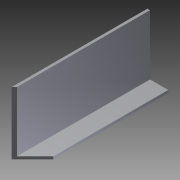
# Autodesk Inventor part: frame corner L 1 by 3
Saved by Autodesk Inventor 2012 (Build 160160000, 160)
## iProperties
Created: 2013-08-08
Part Number: frame corner L 1 by 3
Material: Default
Document SubType Name: Modeling
Designer: Bryce
Density: 1 g/cm^3
Author: Bryce
Autodesk Inventor part; units mm, degrees
ref_plane "YZ Plane" through (0, 0, 0) normal (1, 0, 0) x (0, 1, 0)
ref_plane "XZ Plane" through (0, 0, 0) normal (0, 1, 0) x (-1, 0, 0)
ref_plane "XY Plane" through (0, 0, 0) normal (0, 0, 1) x (1, 0, 0)
sketch "Sketch1" plane through (0, 0, 0) normal (0, 0, 1) x (1, 0, 0)
  line L0 (0, 0) -> (25.4, 0)
  line L1 (25.4, 0) -> (25.4, 3.175)
  line L2 (3.175, 76.2) -> (0, 76.2)
  line L3 (0, 76.2) -> (0, 0)
  line L4 (3.175, 3.175) -> (25.4, 3.175)
  line L5 (3.175, 76.2) -> (3.175, 3.175)
  dimension "d0" = 3.175
  dimension "d1" = 76.2
  dimension "d2" = 25.4
  constraints: 12 end point, 3 perpendicular, 2 horizontal, 2 parallel
  measures "d0" distance of L2.start L2.end
  measures "d1" distance of L2.end L0.start
  measures "d2" distance of L0.start L0.end
extrude "Extrusion1" add sketch "Sketch1" along normal blind 165.1
sketch "Sketch2" plane through (0, 0, 0) normal (0, -1, 0) x (1, 0, 0)
  line L0 (25.4, 165.1) -> (0, 165.1) projected
  line L1 (25.4, 0) -> (25.4, 165.1) projected
  line L2 (0, 165.1) -> (25.4, 139.7)
  dimension "d5" = 45
  constraints: 2 end point, 1 point on line
  measures "d5" angle of L0 L2
extrude "Extrusion2" cut sketch "Sketch2" against normal through all
body "Solid1"
